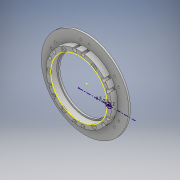
# Autodesk Inventor part: rotor-case
Saved by Autodesk Inventor 2018 (Build 220112000, 112)
## iProperties
Created: 2024-05-26
Part Number: rotor-case
Material: Generic
Document SubType Name: Modeling
Designer: neo
Density: 1 g/cm^3
Appearance: Default
Author: neo
Autodesk Inventor part; units mm, degrees
ref_plane "YZ Plane" through (0, 0, 0) normal (1, 0, 0) x (0, 1, 0)
ref_plane "XZ Plane" through (0, 0, 0) normal (0, 1, 0) x (-1, 0, 0)
ref_plane "XY Plane" through (0, 0, 0) normal (0, 0, 1) x (1, 0, 0)
sketch "Sketch2" plane through (0, 0, 0) normal (1, 0, 0) x (0, 1, 0)
  line L0 (18.4798, 0) -> (-23.1628, 0)
  line L1 (0, 0) -> (-11, 0) construction
  line L2 (-11, 0) -> (-11, -50) construction
  line L3 (-11, -50) -> (0, -50) construction
  line L4 (0, -50) -> (0, 0) construction
  line L5 (0.7575, -40) -> (-11, -40) construction
  line L6 (35.6298, -95) -> (-28.9625, -95) construction
  line L7 (0, -50) -> (-11, -50)
  line L8 (-11, -50) -> (-11, -58)
  line L9 (-11, -58) -> (0, -58)
  line L10 (0, -58) -> (0, -50)
  line L11 (3, -47.5) -> (0, -47.5)
  line L12 (0, -47.5) -> (0, -77.5)
  line L13 (0, -77.5) -> (3, -77.5)
  line L14 (3, -77.5) -> (3, -47.5)
  dimension "d9" = 100
  dimension "d10" = 11
  dimension "d11" = 10
  dimension "d12" = 190
  dimension "d13" = 8
  dimension "d14" = 2.5
  dimension "d15" = 3
  dimension "d16" = 30
  constraints: 30 end point, 6 parallel, 5 horizontal, 4 perpendicular, 1 point on line
  measures "d9" diameter of L3 L0
  measures "d10" distance of L2.end L3.end
  measures "d11" distance between parallel lines of L3 L5
  measures "d12" diameter of L6 L0
  measures "d13" distance of L7.end L8.end
  measures "d14" distance between parallel lines of L3 L11
  measures "d15" distance of L12.end L13.end
  measures "d16" distance of L13.end L11.start
revolve "Revolution3" add sketch "Sketch2" angle 360 about axis through (0, 18.4798, 0) along (0, -1, 0)
sketch "Sketch3" plane through (0, -11, 0) normal (0, -1, 0) x (1, 0, 0)
  circle A0 centre (0, 0) radius 50 projected
  line L0 (0, 0) -> (103.1518, 0)
  circle A1 centre (52.25, 0) radius 4.75
  circle A2 centre (52.25, 0) radius 1.6
  arc A3 (46.338, -10.4421) -> (45.9796, 11.9216) centre (0, 0) ccw construction
  dimension "d19" = 9.5
  dimension "d20" = 3.2
  dimension "d25" = 2.5
  constraints: 3 centre point, 2 coincident, 2 end point, 2 point on circle, 1 horizontal, 1 point on line, 1 tangent
  measures "d19" diameter of A1
  measures "d20" diameter of A2
  measures "d25" radial gap between concentric circles of A0 A3
extrude "Extrusion1" cut sketch "Sketch3" against normal through all contours A2 L0 | L0 A2
extrude "Extrusion2" cut sketch "Sketch3" against normal blind 1 contours L0 A1 A0 | L0 A2 A1 A0 | A0 A1 L0 | A0 A1 L0 A2
pattern_circular "Circular Pattern1" count 6 over 360 about axis through (0, 1.5, 0) along (0, -1, 0) of "Extrusion1", "Extrusion2"
sketch "Sketch4" plane through (0, 3, 0) normal (0, 1, 0) x (1, 0, 0)
  point P0 (0, 0)
sketch "Sketch5" plane through (0, 3, 0) normal (0, 1, 0) x (1, 0, 0)
  circle A0 centre (0, 0) radius 47.5 projected
  line L0 (0, 0) -> (0, 79.7699)
  circle A1 centre (-7.5, 55) radius 1.6
  line L1 (0, 0) -> (104.7189, 0)
  circle A2 centre (-7.5, 65) radius 1.6
  circle A3 centre (7.5, 55) radius 1.6
  circle A4 centre (7.5, 65) radius 1.6
  dimension "d29" = 3.2
  dimension "t" = 7.5
  dimension "d31" = 55
  dimension "d34" = 10
  dimension "d37" = 15
  constraints: 4 centre point, 4 end point, 2 horizontal, 2 vertical, 6 other
  measures "d29" diameter of A1
  measures "t" horizontal distance of point (0, 0) A1.centre
  measures "d31" vertical distance of point (0, 0) A1.centre
  measures "d34" distance of A1.centre A2.centre
  measures "d37" distance of A1.centre A3.centre
extrude "Extrusion3" cut sketch "Sketch5" against normal through all contours A1 | A2 | A3 | A4
pattern_circular "Circular Pattern2" count 6 over 360 about axis through (0, 1.5, 0) along (0, -1, 0) of "Extrusion3"
sketch "Sketch6" plane through (0, -11, 0) normal (0, -1, 0) x (1, 0, 0)
  circle A0 centre (43.8814, -33.9952) radius 1.6 projected
  circle A1 centre (51.3814, -21.0048) radius 1.6 projected
  circle A2 centre (43.8814, -33.9952) radius 3.25
  circle A3 centre (51.3814, -21.0048) radius 3.25
  point P0 (0, 0)
  dimension "d45" = 6.5
  dimension "d46" = 6.5
  constraints: 2 centre point, 2 coincident
  measures "d45" diameter of A2
  measures "d46" diameter of A3
extrude "Extrusion4" cut sketch "Sketch6" against normal up to surface (11 mm away)
pattern_circular "Circular Pattern3" count 6 over 360 about axis through (0, -5.5, 0) along (0, -1, 0) of "Extrusion4"
equation "\"d37\" = 2 * t"
body "Solid2"
